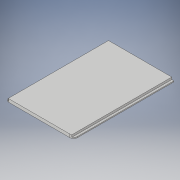
# Autodesk Inventor part: Capstone Calculator Back Cover
Saved by Autodesk Inventor 2018 (Build 220112000, 112)
## iProperties
Created: 2019-09-21
Part Number: Capstone Calculator Back Cover
Material: Generic
Document SubType Name: Modeling
Designer: Hyperspin
Density: 1 g/cm^3
Appearance: Default
Author: Hyperspin
Autodesk Inventor part; units mm, degrees
ref_plane "YZ Plane" through (0, 0, 0) normal (1, 0, 0) x (0, 1, 0)
ref_plane "XZ Plane" through (0, 0, 0) normal (0, 1, 0) x (-1, 0, 0)
ref_plane "XY Plane" through (0, 0, 0) normal (0, 0, 1) x (1, 0, 0)
sketch "Sketch1" plane through (0, 0, 0) normal (0, 0, 1) x (1, 0, 0)
  line L0 (-2.7585, 21.5) -> (79.762, 21.5)
  line L1 (79.762, 23.5) -> (79.762, 25.5)
  line L2 (79.762, 25.5) -> (-2.7585, 25.5)
  line L3 (-2.7585, 25.5) -> (-2.7585, 23.5)
  line L4 (-2.7585, 21.5) -> (-4.7585, 21.5)
  line L5 (-4.7585, 21.5) -> (-4.7585, 23.5)
  line L6 (-4.7585, 23.5) -> (-2.7585, 23.5)
  line L7 (-2.7585, 23.5) -> (-2.7585, 21.5)
  line L8 (79.762, 25.5) -> (-2.7585, 25.5)
  line L9 (81.762, 23.5) -> (79.762, 23.5)
  line L10 (79.762, 21.5) -> (81.762, 21.5)
  line L11 (81.762, 21.5) -> (81.762, 23.5)
  point P0 (0, 0)
  point P1 (2.8, 2)
  dimension "d0" = 4
  dimension "d1" = 2
  dimension "d2" = 2
  constraints: 24 end point, 4 parallel, 2 horizontal, 2 perpendicular
  measures "d0" distance between parallel lines of L0 L2
  measures "d1" distance of L0.start L4.end
  measures "d2" distance of L4.end L5.end
extrude "Extrusion1" add sketch "Sketch1" along normal blind 128.3462
sketch "Sketch3" plane through (-4.7585, 21.5, 0) normal (0, -1, 0) x (1, 0, 0)
  line L0 (0, 128.3462) -> (86.5205, 128.3462) projected
  arc A0 (3.175, 128.3462) -> (0, 125.1712) centre (3.175, 125.1712) ccw
  arc A1 (86.5205, 123.3462) -> (81.5205, 128.3462) centre (81.5205, 123.3462) ccw
  line L1 (0, 0) -> (0, 128.3462) projected
  line L2 (0, 128.3462) -> (3.175, 128.3462)
  line L3 (0, 128.3462) -> (0, 125.1712)
  line L4 (81.5205, 128.3462) -> (86.5205, 128.3462)
  line L5 (86.5205, 128.3462) -> (86.5205, 123.3462)
  point P0 (4.7585, 0)
  dimension "d5" = 3.175
  dimension "d6" = 5
  constraints: 8 end point, 4 point on circle, 2 centre point, 2 perpendicular, 1 tangent
  measures "d5" radius of A0
  measures "d6" radius of A1
extrude "Extrusion2" cut sketch "Sketch3" along normal mid plane 128.3462
sketch "Sketch4" plane through (79.762, 23.5, 127.3462) normal (0, 1, 0) x (1, 0, 0)
  line L0 (-84.5205, 127.3462) -> (-84.5205, 2.175) projected
  line L1 (-82.5205, 127.3462) -> (-82.5205, -0.7746) projected
  line L2 (0, 127.3462) -> (0, 0) projected
  line L3 (2, 127.3462) -> (2, 4) projected
  line L4 (2, 127.3462) -> (0, 127.3462) projected
  line L5 (-82.5205, 127.3462) -> (-84.5205, 127.3462) projected
  arc A0 (-84.5205, 2.175) -> (-82.5205, -0.7746) centre (-81.3455, 2.175) ccw projected
  arc A1 (0, 0) -> (2, 4) centre (-3, 4) ccw projected
  line L6 (-82.5205, 127.3462) -> (-82.5205, -0.7746) projected
  line L7 (-82.5205, 127.3462) -> (-81.7705, 127.3462)
  line L8 (-81.7705, 127.3462) -> (-81.7705, -1)
  line L9 (-81.7705, -1) -> (-82.5205, -1)
  line L10 (-82.5205, -1) -> (-82.5205, -0.7746)
  line L11 (0, 127.3462) -> (-0.75, 127.3462)
  line L12 (-0.75, 127.3462) -> (-0.75, -1)
  line L13 (-0.75, -1) -> (0, -1)
  line L14 (0, -1) -> (0, 0)
  point P0 (-79.762, 127.3462)
  dimension "d9" = 0.75
  dimension "d10" = 0.75
  constraints: 16 end point, 4 parallel, 2 horizontal, 2 perpendicular, 2 point on circle
  measures "d9" distance of L8.end L9.end
  measures "d10" distance of L12.end L13.end
extrude "Extrusion3" cut sketch "Sketch4" against normal blind 0.75 and the other way blind 25.4
sketch "Sketch5" plane through (-4.7585, 21.5, 0) normal (0, -1, 0) x (1, 0, 0)
  line L0 (33.02, 122.7582) -> (53.5005, 122.7582)
  line L1 (53.5005, 122.7582) -> (53.5005, 119.7582)
  line L2 (53.5005, 119.7582) -> (33.02, 119.7582)
  line L3 (33.02, 119.7582) -> (33.02, 122.7582)
  line L4 (3.175, 128.3462) -> (81.5205, 128.3462) projected
  line L5 (86.5205, 0) -> (86.5205, 123.3462) projected
  line L6 (0, 0) -> (0, 125.1712) projected
  point P0 (4.7585, 0)
  dimension "d15" = 5.588
  dimension "d16" = 33.02
  dimension "d17" = 33.02
  dimension "d18" = 3
  constraints: 8 end point, 2 parallel, 1 horizontal, 1 perpendicular
  measures "d15" distance between parallel lines of L0 L4
  measures "d16" distance between parallel lines of L5 L1
  measures "d17" distance between parallel lines of L3 L6
  measures "d18" distance of L0.end L1.end
extrude "Extrusion4" add sketch "Sketch5" along normal blind 1
sketch "Sketch6" plane through (-4.7585, 21.5, 0) normal (0, -1, 0) x (1, 0, 0)
  line L0 (0, 0) -> (0, 125.1712) projected
  line L1 (83.7705, 127.8113) -> (83.7705, 0) projected
  line L2 (83.7705, 0) -> (2.75, 0) projected
  line L3 (2.75, 0) -> (2.75, 128.3176) projected
  arc A0 (3.175, 128.3462) -> (2.75, 128.3176) centre (3.175, 125.1712) ccw projected
  line L4 (81.5205, 128.3462) -> (3.175, 128.3462) projected
  arc A1 (83.7705, 127.8113) -> (81.5205, 128.3462) centre (81.5205, 123.3462) ccw projected
  line L5 (6.75, 70.3822) -> (6.75, 114.3462)
  line L6 (0, 0) -> (86.5205, 0) projected
  line L7 (6.75, 114.3462) -> (79.7705, 114.3462)
  line L8 (79.7705, 114.3462) -> (79.7705, 0)
  line L9 (79.7705, 0) -> (6.75, 0)
  line L10 (6.75, 0) -> (6.75, 114.3462)
  point P0 (4.7585, 0)
  dimension "d21" = 4
  dimension "d22" = 14
  dimension "d23" = 4
  constraints: 10 end point, 2 parallel, 1 horizontal, 1 perpendicular, 1 point on line, 1 vertical
  measures "d21" distance between parallel lines of L3 L5
  measures "d22" distance from line of L5.end L4
  measures "d23" distance between parallel lines of L1 L8
extrude "Extrusion5" cut sketch "Sketch6" against normal blind 1.75 contours L2 L10 L5 L7 L8
body "Solid1"
